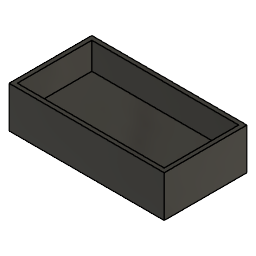
koszyk_na_baterie (Autodesk Fusion 360 design; units mm, degrees)
part number: 2025-11-20-20-18-58-786
part number: 2025-11-29-21-09-07-415
Autodesk Fusion 360 part; units mm, degrees
note: some values were not read from the file. Set by a fixed rule: which face or edge a step refers to.
sketch "Szkic1" plane through (0, 0, 0) normal (0, 0, 1) x (1, 0, 0)
  line L0 (0, 0) -> (75, 0)
  line L1 (75, 0) -> (75, 40)
  line L2 (75, 40) -> (0, 40)
  line L3 (0, 40) -> (0, 0)
  dimension "d1" = 75
  dimension "d2" = 40
  constraint horizontal L0
  constraint vertical L1
  constraint horizontal L2
  constraint vertical L3
  constraint coincident L0.start L3.end
  measures "d1" distance of L0.start L0.end
  measures "d2" distance of L0.start L2.end
extrude "Wyciągnięcie proste1" add sketch "Szkic1" along normal blind 20 makes body 1
shell "Skorupa1" thickness 2 removed faces 1 at (25, 26.6667, 20) on bodies 1
extrude "Wyciągnięcie proste2" add 1 faces at (25.6667, 14, 2) along direction (0, 0, 1) blind 5 on bodies 1 bodies 1
copy_body "Bryła->Komponent1" bodies 1 removing the originals makes body 2 in component "koszyk"
component "koszyk" placed x (1, 0, 0) y (0, 1, 0) z (0, 0, 1) at (0, 0, 0)
named bodies: "koszyk"
